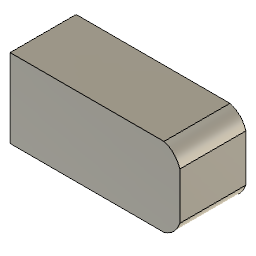
ai_robo (Autodesk Fusion 360 design; units mm, degrees)
part number: 2025-10-12-23-10-22-263
Autodesk Fusion 360 part; units mm, degrees
sketch "スケッチ1" plane through (0, 0, 0) normal (0, 1, 0) x (1, 0, 0)
  line L0 (-48.05, -22.3) -> (-4.5, -22.3)
  line L1 (0, -17.8) -> (0, -4.5)
  line L2 (-4.5, 0) -> (-48.05, 0)
  line L3 (-48.05, 0) -> (-48.05, -22.3)
  line L4 (0, -13.65) -> (5, -13.65)
  line L5 (5, -13.65) -> (5, -8.65)
  line L6 (5, -8.65) -> (0, -8.65)
  line L7 (0, -8.65) -> (0, -13.65)
  spline S0 degree 5 poles (-4.5, 0) (-4.1761, -0.0977) (-3.551, -0.3263) (-2.6815, -0.7689) (-1.692, -1.538) (-0.8859, -2.5754) (-0.394, -3.5009) (-0.1187, -4.1718) (0, -4.5) knots 0 0 0 0 0 0 0.1 0.2 0.3 0.387808 0.387808 0.387808 0.387808 0.387808 0.387808
  line L8 (-0.2882, -3.7033) -> (0.2882, -5.2967)
  spline S1 degree 5 poles (-4.5, -22.3) (-4.1747, -22.2035) (-3.5471, -21.9766) (-2.6744, -21.534) (-1.6867, -20.7645) (-0.8818, -19.7232) (-0.3911, -18.7948) (-0.117, -18.1241) (0, -17.8) knots 0 0 0 0 0 0 0.1 0.2 0.3 0.38591 0.38591 0.38591 0.38591 0.38591 0.38591
  line L9 (-0.2891, -18.6007) -> (0.2891, -16.9993)
  dimension "d3" = 5
  dimension "d4" = 5
  dimension "d6" = 4.5
  dimension "d7" = 4.5
  constraint horizontal L0
  constraint vertical L1
  constraint horizontal L2
  constraint vertical L3
  constraint horizontal L4
  constraint vertical L5
  constraint horizontal L6
  constraint vertical L7
  constraint coincident L1 L4.start
  constraint midpoint L1.end L8
  constraint coincident L0.end S1.start
  constraint coincident L1.start S1.end
  constraint midpoint L1.start L9
  measures "d3" distance of L4.start L4.end
  measures "d4" distance of L4.end L5.end
  measures "d6" distance of origin L2.start
  measures "d7" distance of origin L1.end
extrude "押し出し1" add sketch "スケッチ1" along normal blind 18.7 contours L0 L1 L2 L3 L7 S0 S1
